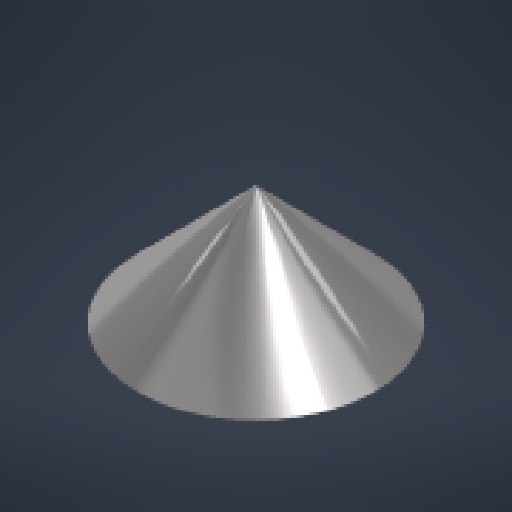
# Autodesk Inventor part: Kathode
Saved by Autodesk Inventor 2025 (Build 290162000, 162)
## iProperties
Created: 2025-01-24
Part Number: Kathode
Material: Сталь, легированная
Document SubType Name: Modeling
Designer: khrip
Density: 7.73 g/cm^3
Appearance: С умеренной полировкой
Author: khrip
Autodesk Inventor part; units mm, degrees
ref_plane "YZ Plane" through (0, 0, 0) normal (1, 0, 0) x (0, 1, 0)
ref_plane "XZ Plane" through (0, 0, 0) normal (0, 1, 0) x (-1, 0, 0)
ref_plane "XY Plane" through (0, 0, 0) normal (0, 0, 1) x (1, 0, 0)
sketch "Эскиз1" plane through (0, 0, 0) normal (0, 0, 1) x (1, 0, 0)
  line L0 (0, 0) -> (0, -22.4194)
  line L1 (0, 0) -> (7.0711, -7.0711)
  line L2 (7.0711, -7.0711) -> (7.1771, -6.965)
  line L3 (7.1771, -6.965) -> (0.1061, 0.1061)
  line L4 (0.1061, 0.1061) -> (0, 0)
  line L5 (0, 0) -> (10, 0) construction
  line L6 (7.0711, -7.0711) -> (7.7782, -7.7782)
  line L7 (7.7782, -7.7782) -> (14.8492, -14.8492)
  line L8 (14.8492, -14.8492) -> (14.9553, -14.7432)
  line L9 (14.9553, -14.7432) -> (7.8842, -7.6721)
  line L10 (7.8842, -7.6721) -> (7.7782, -7.7782)
  dimension "d0" = 10
  dimension "d1" = 45
  dimension "d2" = 0.15
  dimension "d4" = 1
  dimension "d5" = 10
  dimension "d6" = 0.15
  constraints: 22 end point, 4 parallel, 2 perpendicular, 1 equal length, 1 horizontal, 1 vertical
  measures "d0" distance of L0.start L1.end
  measures "d1" angle of L1 L5
  measures "d2" distance of L2.end L1.end
  measures "d4" distance of L1.end L6.end
  measures "d5" distance of L7.start L7.end
  measures "d6" distance of L8.end L7.end
revolve "Вращение1" add sketch "Эскиз1" angle 360 about axis through (0, 0, 0) along (0, -1, 0) contours L4 L3 L2 L1
